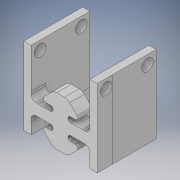
# Autodesk Inventor part: Actual
Saved by Autodesk Inventor 2018 (Build 220112000, 112)
## iProperties
Created: 2018-03-23
Part Number: Actual
Material: Generic
Document SubType Name: Modeling
Designer: Student
Density: 1 g/cm^3
Appearance: Default
Author: Student
Autodesk Inventor part; units mm, degrees
ref_plane "YZ Plane" through (0, 0, 0) normal (1, 0, 0) x (0, 1, 0)
ref_plane "XZ Plane" through (0, 0, 0) normal (0, 1, 0) x (-1, 0, 0)
ref_plane "XY Plane" through (0, 0, 0) normal (0, 0, 1) x (1, 0, 0)
sketch "Sketch3" plane through (0, 0, 0) normal (0, 0, 1) x (1, 0, 0)
  line L0 (-5.4704, -4.1494) -> (-2.243, -0.9279)
  arc A0 (0, 0) -> (-2.243, -0.9279) centre (0, -3.175) ccw
  line L1 (0, 0) -> (3.4185, 0)
  arc A1 (5.6615, -0.9279) -> (3.4185, 0) centre (3.4185, -3.175) ccw
  line L2 (5.6615, -0.9279) -> (8.8889, -4.1494)
  arc A2 (8.1257, -5.9944) -> (8.8889, -4.1494) centre (8.1257, -4.914) ccw
  line L3 (8.1257, -5.9944) -> (5.9968, -5.9944)
  arc A3 (5.9968, -5.9944) -> (4.9478, -7.0434) centre (5.9968, -7.0434) ccw
  arc A4 (4.9478, -7.1552) -> (5.9968, -8.2042) centre (5.9968, -7.1552) ccw
  line L4 (4.9478, -7.0434) -> (4.9478, -7.1552)
  arc A5 (-1.5292, -7.0434) -> (-2.5783, -5.9944) centre (-2.5783, -7.0434) ccw
  line L5 (-2.5783, -5.9944) -> (-4.7072, -5.9944)
  arc A6 (-5.4704, -4.1494) -> (-4.7072, -5.9944) centre (-4.7072, -4.914) ccw
  arc A7 (-2.5783, -8.2042) -> (-1.5292, -7.1552) centre (-2.5783, -7.1552) ccw
  line L6 (-1.5292, -7.1552) -> (-1.5292, -7.0434)
  line L7 (-3.6079, -8.2042) -> (-2.5783, -8.2042)
  line L8 (5.9968, -8.2042) -> (7.0264, -8.2042)
  line L9 (-7.8411, -8.2042) -> (-4.6239, -8.2042)
  line L10 (8.0424, -8.2042) -> (11.2597, -8.2042)
  line L11 (-3.6079, -8.2042) -> (-4.6239, -8.2042)
  line L12 (8.0424, -8.2042) -> (11.2597, -8.2042)
  line L13 (7.0264, -8.2042) -> (8.0424, -8.2042)
  line L14 (1.7093, 4.4958) -> (1.7093, -14.4322)
  line L15 (-8.8571, -8.204) -> (-7.8411, -8.2042)
  line L16 (11.2597, -8.2042) -> (11.2597, -8.2042)
  arc A8 (-10.9906, -6.0706) -> (-8.8571, -8.204) centre (-8.8825, -6.096) ccw
  arc A9 (-10.9906, -6.0706) -> (-8.8571, -8.204) centre (-8.8825, -6.096) ccw
  line L17 (-10.9907, -5.0546) -> (-10.9906, -6.0706)
  line L18 (-10.9907, 12.258) -> (-10.9907, -5.0546)
  line L19 (-10.9907, -5.0546) -> (-10.9907, 12.258)
  line L20 (-11.2451, -10.6176) -> (1.7093, -10.6176)
  line L21 (14.4093, 12.258) -> (17.5843, 12.258)
  line L22 (14.4093, -5.0546) -> (14.4091, -6.0706)
  line L23 (14.4093, 12.258) -> (14.4093, -5.0546)
  arc A10 (12.2757, -8.204) -> (14.4091, -6.0706) centre (12.3011, -6.096) ccw
  line L24 (12.2757, -8.204) -> (11.2597, -8.2042)
  line L25 (11.2597, -8.2042) -> (8.0424, -8.2042)
  line L26 (7.0264, -8.2042) -> (8.0424, -8.2042)
  line L27 (14.6636, -10.6176) -> (1.7093, -10.6176)
  arc A11 (-10.9907, 12.258) -> (-10.9907, 12.258) centre (-10.9907, 11.75) ccw
  line L28 (-14.1657, 12.258) -> (-10.9907, 12.258)
  line L29 (14.6636, -10.6176) -> (17.5843, -10.6176)
  line L30 (-11.2451, -10.6176) -> (-14.1657, -10.6176)
  line L31 (-14.1657, 12.258) -> (-14.1657, -10.6176)
  line L32 (17.5843, 12.258) -> (17.5843, -10.6176)
  point P0 (0, 0)
  dimension "d8" = 3.175
  constraints: 66 end point, 24 point on circle, 12 centre point, 8 symmetric about line, 5 horizontal, 2 point on line, 2 vertical, 1 coincident, 1 perpendicular, 1 other
  measures "d8" distance of L28.start L19.end
extrude "Extrusion1" add sketch "Sketch3" along normal blind 6.35 contours L0 A0 L1 L14 L20 L30 L31 L28 A11 L18 L17 A8 L15 L9 L11 L7 A7 L6 A5 L5 A6 | L1 A1 L2 A2 L3 A3 L4 A4 L8 L13 L10 L24 A10 L22 L23 L21 L32 L29 L27 L14 | L18 A11 picked at (-11.1588, 11.7704)
mirror "Mirror1" about plane through (-14.1657, -10.6176, 0) normal (0, -1, 0) of "Extrusion1"
sketch "Sketch9" plane through (0, 0, 6.35) normal (0, 0, 1) x (1, 0, 0)
  line L0 (-14.1657, 12.258) -> (-14.1657, -33.4932) projected
  line L1 (-14.1657, -21.2352) -> (-10.9907, -21.2352)
  line L2 (-10.9907, -16.1806) -> (-10.9907, -33.4932) projected
  line L3 (3.4185, 0) -> (0, 0) projected
  line L4 (1.7093, 0) -> (1.7093, -21.2352)
  line L5 (17.5843, -21.2352) -> (14.4093, -21.2352)
  line L6 (-10.9907, -33.4932) -> (-14.1657, -33.4932) projected
  line L7 (14.4093, -33.4932) -> (14.4093, -16.1806) projected
  line L8 (17.5843, 12.258) -> (17.5843, -33.4932) projected
  line L9 (17.5843, -33.4932) -> (14.4093, -33.4932) projected
  point P0 (0, -21.2352)
  constraints: 6 end point, 2 point on line, 2 symmetric about line, 1 midpoint, 1 vertical
extrude "Extrusion5" cut sketch "Sketch9" against normal through all
sketch "Sketch10" plane through (0, 0, 0) normal (0, 0, -1) x (-1, 0, 0)
  line L0 (-17.5843, 12.258) -> (-14.4093, 12.258) projected
  line L1 (-17.5843, 12.258) -> (-17.5843, -21.2352) projected
  line L2 (-14.4093, 12.258) -> (-14.4093, -5.0546) projected
  line L3 (-14.4093, -21.2352) -> (-14.4093, -16.1806) projected
  line L4 (-14.4093, -5.0546) -> (-14.4091, -6.0706) projected
  line L5 (-14.4093, -5.0546) -> (-14.4093, -16.1806)
  line L6 (-17.5843, -21.2352) -> (-14.4093, -21.2352) projected
  line L7 (-3.4185, 0) -> (0, 0) projected
  line L8 (-1.7093, 0) -> (-1.7093, -21.2352)
  line L9 (-3.4185, -21.2352) -> (0, -21.2352) projected
  line L10 (14.1657, 12.258) -> (10.9907, 12.258)
  line L11 (14.1657, 12.258) -> (14.1657, -21.2352)
  line L12 (10.9907, 12.258) -> (10.9907, -5.0546)
  line L13 (10.9907, -21.2352) -> (10.9907, -16.1806)
  line L14 (10.9907, -5.0546) -> (10.9906, -6.0706)
  line L15 (10.9907, -5.0546) -> (10.9907, -16.1806)
  line L16 (14.1657, -21.2352) -> (10.9907, -21.2352)
  constraints: 18 end point, 7 symmetric about line, 2 midpoint, 1 vertical
extrude "Extrusion6" add sketch "Sketch10" along normal blind 19.05
sketch "Sketch11" plane through (17.5843, -21.2352, 6.35) normal (1, 0, 0) x (0, 0, -1)
  line L0 (6.35, 33.4932) -> (0, 33.4932) projected
  line L1 (6.35, 33.4932) -> (25.4, 33.4932) projected
  line L2 (0, 33.4932) -> (0, 0) projected
  line L3 (0, 0) -> (6.35, 0) projected
  line L4 (6.35, 0) -> (25.4, 0) projected
  line L5 (25.4, 33.4932) -> (25.4, 0) projected
  line L6 (0, 33.4932) -> (0, 29.6832) construction
  line L7 (0, 33.4932) -> (3.81, 33.4932) construction
  line L8 (6.35, 33.4932) -> (0, 33.4932) construction
  circle A0 centre (3.81, 29.6832) radius 2.54
  line L9 (25.4, 33.4932) -> (0, 33.4932) construction
  line L10 (12.7, 33.4932) -> (12.7, -0.3968)
  circle A1 centre (21.59, 29.6832) radius 2.54
  point P0 (6.35, 21.2352)
  dimension "d26" = 3.81
  dimension "d27" = 3.81
  dimension "d28" = 5.08
  constraints: 6 end point, 2 centre point, 2 point on line, 1 horizontal alignment, 1 midpoint, 1 perpendicular, 1 symmetric about line, 1 vertical alignment, 1 other
  measures "d26" distance of L0.end L6.end
  measures "d27" distance of L0.end L7.end
  measures "d28" diameter of A0
extrude "Extrusion7" cut sketch "Sketch11" against normal through all contours A0 | A1
body "Solid1"
